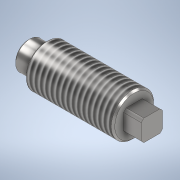
# Autodesk Inventor part: 10-螺杆
Saved by Autodesk Inventor 2022 (Build 260153000, 153)
## iProperties
Created: 2023-01-10
Part Number: 10-螺杆
Material: 不锈钢
Document SubType Name: Modeling
Designer: Lzy18
Density: 8 g/cm^3
Appearance: 半抛光
Author: Lzy18
Autodesk Inventor part; units mm, degrees
ref_plane "YZ Plane" through (0, 0, 0) normal (1, 0, 0) x (0, 1, 0)
ref_plane "XZ Plane" through (0, 0, 0) normal (0, 1, 0) x (-1, 0, 0)
ref_plane "XY Plane" through (0, 0, 0) normal (0, 0, 1) x (1, 0, 0)
sketch "草图1" plane through (0, 0, 0) normal (0, 0, 1) x (1, 0, 0)
  line L0 (0, 0) -> (10, 0)
  line L1 (10, 0) -> (10, -8)
  line L2 (10, -8) -> (0, -8)
  line L3 (0, -8) -> (0, 0)
  line L4 (10, 0) -> (60, 0)
  line L5 (60, 0) -> (60, -12)
  line L6 (60, -12) -> (10, -12)
  line L7 (10, -12) -> (10, 0)
  dimension "d0" = 10
  dimension "d1" = 8
  dimension "d2" = 50
  dimension "d3" = 12
  constraints: 16 end point, 4 parallel, 2 horizontal, 2 perpendicular
  measures "d0" distance of L1.end L2.end
  measures "d1" distance of L0.end L1.end
  measures "d2" distance of L5.end L6.end
  measures "d3" distance of L4.end L5.end
revolve "旋转1" add sketch "草图1" angle 360 about axis through (10, 0, 0) along (1, 0, 0)
chamfer "倒角1" distance 1 angle 45 1 edges at (60, 12, 0)
chamfer "倒角2" distance 1 angle 45 1 edges at (0, 8, 0)
chamfer "倒角3" distance 1 angle 45 1 edges at (10, 12, 0)
sketch "草图2" plane through (60, 0, 0) normal (1, 0, 0) x (0, 0, -1)
  line L0 (-4.5, 6) -> (4.5, 6)
  line L1 (6, 4.5) -> (6, -4.5)
  line L2 (4.5, -6) -> (-4.5, -6)
  line L3 (-6, -4.5) -> (-6, 4.5)
  line L4 (-6, 6) -> (6, -6) construction
  line L5 (6, 6) -> (-6, -6) construction
  arc A0 (-4.5, 6) -> (-6, 4.5) centre (0, 0) ccw
  arc A1 (-6, -4.5) -> (-4.5, -6) centre (0, 0) ccw
  arc A2 (4.5, -6) -> (6, -4.5) centre (0, 0) ccw
  arc A3 (6, 4.5) -> (4.5, 6) centre (0, 0) ccw
  dimension "d15" = 12
  dimension "d16" = 12
  constraints: 12 end point, 8 point on circle, 4 centre point, 2 midpoint, 2 parallel, 1 coincident, 1 horizontal, 1 perpendicular
  measures "d15" distance of L4.end L5.end
  measures "d16" distance of L5.start L4.end
extrude "拉伸1" add sketch "草图2" along normal blind 10
thread "螺纹1" size "M24x3" designation "M24" class "6g" standard "GB Metric profile" length 48
